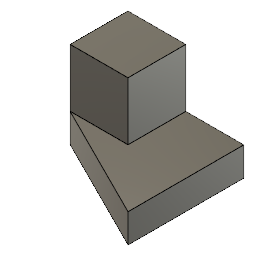
3DD1 (Autodesk Fusion 360 design; units mm, degrees)
Autodesk Fusion 360 part; units mm, degrees
sketch "Sketch1" plane through (0, 0, 0) normal (0, 1, 0) x (1, 0, 0)
  line L0 (0, 0) -> (40, 0)
  line L1 (40, 0) -> (40, -40)
  line L2 (40, -40) -> (0, -20)
  line L3 (0, -20) -> (0, 0)
  dimension "d1" = 40
  dimension "d2" = 20
  dimension "d3" = 40
extrude "Extrude1" add sketch "Sketch1" along normal blind 10
sketch "Sketch2" plane through (0, 10, 0) normal (0, 1, 0) x (-1, 0, 0)
  line L0 (0, 20) -> (-40, 40)
  line L1 (-40, 40) -> (-40, 0)
  line L2 (-40, 0) -> (0, 0)
  line L3 (0, 0) -> (0, 20)
  line L4 (0, 0) -> (-20, 0)
  line L5 (0, 0) -> (0, 20)
  line L6 (0, 20) -> (-20, 20)
  line L7 (-20, 20) -> (-20, 0)
  dimension "d6" = 20
  dimension "d7" = 20
extrude "Extrude2" add sketch "Sketch2" along normal blind 20 contours L2 L3 L4 L5 L6 L7
